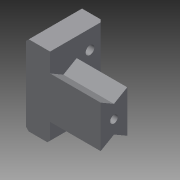
# Autodesk Inventor part: switchlock1l
Saved by Autodesk Inventor 2015 (Build 190159000, 159)
## iProperties
Created: 2020-08-08
Part Number: switchlock1l
Material: 일반
Document SubType Name: Modeling
Designer: penta
Density: 1 g/cm^3
Appearance: 기본값
Author: penta
Autodesk Inventor part; units mm, degrees
ref_plane "YZ Plane" through (0, 0, 0) normal (1, 0, 0) x (0, 1, 0)
ref_plane "XZ Plane" through (0, 0, 0) normal (0, 1, 0) x (-1, 0, 0)
ref_plane "XY Plane" through (0, 0, 0) normal (0, 0, 1) x (1, 0, 0)
sketch "스케치1" plane through (0, 0, 0) normal (0, 1, 0) x (-1, 0, 0)
  line L0 (0, 0) -> (-9, 0)
  line L1 (-9, 0) -> (-9, -30)
  line L2 (-9, -30) -> (0, -30)
  line L3 (0, -30) -> (0, 0)
  dimension "d0" = 9
  dimension "d1" = 30
  constraints: 8 end point, 2 parallel, 1 horizontal, 1 perpendicular
  measures "d0" distance of L2.end L1.end
  measures "d1" distance of L1.end L0.end
extrude "돌출1" add sketch "스케치1" along normal blind 10
sketch "스케치2" plane through (0, 10, 0) normal (0, 1, 0) x (1, 0, 0)
  line L0 (9, 30) -> (0, 30)
  line L1 (0, 0) -> (9, 0)
  line L2 (9, 0) -> (9, 30)
  line L3 (0, 0) -> (0, 2)
  line L4 (0, 28) -> (0, 30)
  line L5 (0, 28) -> (6, 28)
  line L6 (6, 28) -> (6, 2)
  line L7 (6, 2) -> (0, 2)
  dimension "d62" = 6
  constraints: 16 end point, 2 equal length, 2 horizontal, 2 perpendicular, 1 vertical
  measures "d62" distance of L4.start L5.end
extrude "돌출2" add sketch "스케치2" along normal blind 10
hole "구멍1" at (9, 15, -23) direction (-1, 0, 0) diameter 3.25 end through all
hole "구멍2" at (9, 15, -7) direction (-1, 0, 0) diameter 3.25 end through all
sketch "스케치5" plane through (9, 0, 0) normal (1, 0, 0) x (0, 0, -1)
  line L0 (6.8868, 10) -> (9.7735, 5)
  line L1 (9.7735, 5) -> (6.8868, 0)
  line L2 (23.1132, 0) -> (20.2265, 5)
  line L3 (20.2265, 5) -> (23.1132, 10)
  line L4 (6.8868, 0) -> (23.1132, 0)
  line L5 (23.1132, 10) -> (17.6, 10)
  line L6 (17.6, 3.4989) -> (15, 1.9978)
  line L7 (15, 1.9978) -> (12.4, 3.4989)
  line L8 (12.4, 3.4989) -> (12.4, 6.5011)
  line L9 (12.4, 6.5011) -> (15, 8.0022)
  line L10 (15, 8.0022) -> (17.6, 6.5011)
  line L11 (17.6, 6.5011) -> (17.6, 3.4989)
  line L12 (17.6, 6.5011) -> (17.6, 10)
  line L13 (12.4, 6.5011) -> (12.4, 10)
  line L14 (12.4, 10) -> (6.8868, 10)
  line L15 (17.6, 10) -> (12.4, 10)
  point P0 (4, 5)
  point P1 (26, 5)
  point P2 (4, 5)
  point P3 (4, 10)
  point P4 (26, 5)
  point P5 (26, 10)
  point P6 (15, 5)
  point P7 (17.6, 5)
  point P8 (15, 5)
  constraints: 32 end point, 6 perpendicular, 3 coincident, 3 parallel, 1 horizontal, 1 midpoint, 21 other
extrude "돌출5" add sketch "스케치5" along normal blind 16 contours L14 L13 L8 L7 L6 L11 L12 L5 L3 L2 L4 L1 L0
sketch "스케치6" plane through (25, 0, 0) normal (1, 0, 0) x (0, 0, -1)
  line L0 (20.2265, 5) -> (23.1132, 10) projected
  line L1 (23.1132, 10) -> (17.6, 10) projected
  line L2 (17.6, 10) -> (17.6, 3.4989) projected
  line L3 (17.6, 3.4989) -> (15, 1.9978) projected
  line L4 (15, 1.9978) -> (12.4, 3.4989) projected
  line L5 (12.4, 3.4989) -> (12.4, 10) projected
  line L6 (12.4, 10) -> (6.8868, 10) projected
  line L7 (6.8868, 10) -> (9.7735, 5) projected
  line L8 (9.7735, 5) -> (6.8868, 0) projected
  line L9 (6.8868, 0) -> (23.1132, 0) projected
  line L10 (23.1132, 0) -> (20.2265, 5) projected
  line L11 (17.6, 10) -> (12.4, 10)
  point P0 (0, 0)
  constraints: 2 end point, 1 horizontal
extrude "돌출6" add sketch "스케치6" along normal blind 3
hole "구멍4" at (28, 5, -15) direction (-1, 0, 0) diameter 2.85 end up to surface
thicken "두껍게 하기1" operation add thickness 0.5 both sides no extend neighbours yes toward (0, 0, 1) faces at (14.3333, 5.6659, -12.4) (14.3333, 2.4981, -14.1333) (14.3333, 2.9985, -16.7333) (14.3333, 7.833, -17.6)
thicken "두껍게 하기2" operation add thickness 0.2 both sides no extend neighbours yes toward (0, -0.5, -0.8660254) faces at (14.3333, 2.8685, -8.5429) (14.3333, 7.1315, -8.5429) (14.3333, 2.8685, -21.4571) (14.3333, 7.1315, -21.4571)
thicken "두껍게 하기3" operation add thickness 0.1 both sides no extend neighbours yes toward (0, 0, -1) faces at (2, 13.3333, -28) (4, 13.3333, -2)
chamfer "모따기1" distance 1 angle 45 2 edges at (9, 10, -30) (9, 20, -15)
chamfer "모따기2" distance 1 angle 45 2 edges at (0, 10, 0) (0, 10, -30)
